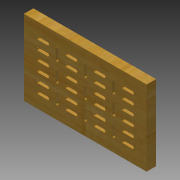
# Autodesk Inventor part: suporte
Saved by Autodesk Inventor 2014 (Build 180170000, 170)
## iProperties
Created: 2015-05-28
Part Number: suporte
Material: Generic
Document SubType Name: Modeling
Designer: Gabriel
Density: 1 g/cm^3
Appearance: Default
Author: Gabriel
Autodesk Inventor part; units mm, degrees
ref_plane "YZ Plane" through (0, 0, 0) normal (1, 0, 0) x (0, 1, 0)
ref_plane "XZ Plane" through (0, 0, 0) normal (0, 1, 0) x (-1, 0, 0)
ref_plane "XY Plane" through (0, 0, 0) normal (0, 0, 1) x (1, 0, 0)
sketch "Sketch1" plane through (0, 0, 0) normal (0, 1, 0) x (-1, 0, 0)
  line L0 (0, 0) -> (130, 0)
  line L1 (130, 0) -> (130, 80)
  line L2 (130, 80) -> (0, 80)
  line L3 (0, 80) -> (0, 0)
  line L4 (0, 0) -> (0, 20)
  line L5 (130, 0) -> (110, 0)
  line L6 (130, 80) -> (110, 80)
  line L7 (0, 80) -> (0, 55)
  line L8 (23.5, 55) -> (25, 55)
  line L9 (25, 55) -> (23.5, 55) construction
  line L10 (25, 56.5) -> (15, 56.5)
  line L11 (15, 53.5) -> (25, 53.5)
  arc A0 (25, 53.5) -> (25, 56.5) centre (25, 55) ccw
  arc A1 (15, 56.5) -> (15, 53.5) centre (15, 55) ccw
  line L12 (20, 25) -> (15, 25)
  line L13 (15, 25) -> (25, 25) construction
  line L14 (15, 23.5) -> (25, 23.5)
  line L15 (25, 26.5) -> (15, 26.5)
  arc A2 (15, 26.5) -> (15, 23.5) centre (15, 25) ccw
  arc A3 (25, 23.5) -> (25, 26.5) centre (25, 25) ccw
  line L16 (20, 55) -> (20, 45)
  line L17 (25, 45) -> (15, 45) construction
  line L18 (25, 46.5) -> (15, 46.5)
  line L19 (15, 43.5) -> (25, 43.5)
  arc A4 (25, 43.5) -> (25, 46.5) centre (25, 45) ccw
  arc A5 (15, 46.5) -> (15, 43.5) centre (15, 45) ccw
  line L20 (25, 35) -> (15, 35) construction
  line L21 (25, 36.5) -> (15, 36.5)
  line L22 (15, 33.5) -> (25, 33.5)
  arc A6 (25, 33.5) -> (25, 36.5) centre (25, 35) ccw
  arc A7 (15, 36.5) -> (15, 33.5) centre (15, 35) ccw
  line L23 (20, 55) -> (20, 65)
  line L24 (20, 65) -> (20, 66.5)
  line L25 (25, 65) -> (15, 65) construction
  line L26 (25, 66.5) -> (15, 66.5)
  line L27 (15, 63.5) -> (25, 63.5)
  arc A8 (25, 63.5) -> (25, 66.5) centre (25, 65) ccw
  arc A9 (15, 66.5) -> (15, 63.5) centre (15, 65) ccw
  line L28 (25, 15) -> (15, 15) construction
  line L29 (25, 16.5) -> (15, 16.5)
  line L30 (15, 13.5) -> (25, 13.5)
  arc A10 (25, 13.5) -> (25, 16.5) centre (25, 15) ccw
  arc A11 (15, 16.5) -> (15, 13.5) centre (15, 15) ccw
  line L31 (20, 80) -> (35, 80)
  line L32 (35, 80) -> (50, 80)
  line L33 (50, 80) -> (70, 80)
  line L34 (70, 80) -> (90, 80)
  line L35 (46.5, 55) -> (45, 55)
  line L36 (45, 55) -> (46.5, 55) construction
  line L37 (45, 56.5) -> (55, 56.5)
  line L38 (55, 53.5) -> (45, 53.5)
  arc A12 (45, 56.5) -> (45, 53.5) centre (45, 55) ccw
  arc A13 (55, 53.5) -> (55, 56.5) centre (55, 55) ccw
  line L39 (50, 25) -> (55, 25)
  line L40 (55, 25) -> (45, 25) construction
  line L41 (55, 23.5) -> (45, 23.5)
  line L42 (45, 26.5) -> (55, 26.5)
  arc A14 (55, 23.5) -> (55, 26.5) centre (55, 25) ccw
  arc A15 (45, 26.5) -> (45, 23.5) centre (45, 25) ccw
  line L43 (45, 45) -> (55, 45) construction
  line L44 (45, 46.5) -> (55, 46.5)
  line L45 (55, 43.5) -> (45, 43.5)
  arc A16 (45, 46.5) -> (45, 43.5) centre (45, 45) ccw
  arc A17 (55, 43.5) -> (55, 46.5) centre (55, 45) ccw
  line L46 (45, 35) -> (55, 35) construction
  line L47 (45, 36.5) -> (55, 36.5)
  line L48 (55, 33.5) -> (45, 33.5)
  arc A18 (45, 36.5) -> (45, 33.5) centre (45, 35) ccw
  arc A19 (55, 33.5) -> (55, 36.5) centre (55, 35) ccw
  line L49 (45, 65) -> (55, 65) construction
  line L50 (45, 66.5) -> (55, 66.5)
  line L51 (55, 63.5) -> (45, 63.5)
  arc A20 (45, 66.5) -> (45, 63.5) centre (45, 65) ccw
  arc A21 (55, 63.5) -> (55, 66.5) centre (55, 65) ccw
  line L52 (45, 15) -> (55, 15) construction
  line L53 (45, 16.5) -> (55, 16.5)
  line L54 (55, 13.5) -> (45, 13.5)
  arc A22 (45, 16.5) -> (45, 13.5) centre (45, 15) ccw
  arc A23 (55, 13.5) -> (55, 16.5) centre (55, 15) ccw
  line L55 (50, 80) -> (65, 80)
  line L56 (65, 80) -> (80, 80)
  arc A24 (75, 56.5) -> (75, 53.5) centre (75, 55) ccw
  line L57 (83.5, 55) -> (85, 55)
  line L58 (85, 55) -> (83.5, 55) construction
  line L59 (75, 53.5) -> (85, 53.5)
  arc A25 (85, 53.5) -> (85, 56.5) centre (85, 55) ccw
  arc A26 (85, 23.5) -> (85, 26.5) centre (85, 25) ccw
  arc A27 (75, 26.5) -> (75, 23.5) centre (75, 25) ccw
  line L60 (75, 23.5) -> (85, 23.5)
  line L61 (75, 43.5) -> (85, 43.5)
  line L62 (85, 45) -> (75, 45) construction
  arc A28 (75, 46.5) -> (75, 43.5) centre (75, 45) ccw
  line L63 (85, 46.5) -> (75, 46.5)
  arc A29 (85, 43.5) -> (85, 46.5) centre (85, 45) ccw
  line L64 (80, 25) -> (75, 25)
  line L65 (85, 36.5) -> (75, 36.5)
  arc A30 (85, 33.5) -> (85, 36.5) centre (85, 35) ccw
  line L66 (85, 35) -> (75, 35) construction
  line L67 (75, 33.5) -> (85, 33.5)
  arc A31 (75, 36.5) -> (75, 33.5) centre (75, 35) ccw
  line L68 (85, 26.5) -> (75, 26.5)
  line L69 (75, 25) -> (85, 25) construction
  line L70 (85, 56.5) -> (75, 56.5)
  line L71 (75, 63.5) -> (85, 63.5)
  line L72 (85, 65) -> (75, 65) construction
  line L73 (85, 66.5) -> (75, 66.5)
  arc A32 (75, 66.5) -> (75, 63.5) centre (75, 65) ccw
  arc A33 (85, 63.5) -> (85, 66.5) centre (85, 65) ccw
  line L74 (85, 16.5) -> (75, 16.5)
  line L75 (85, 15) -> (75, 15) construction
  arc A34 (75, 16.5) -> (75, 13.5) centre (75, 15) ccw
  arc A35 (85, 13.5) -> (85, 16.5) centre (85, 15) ccw
  line L76 (75, 13.5) -> (85, 13.5)
  line L77 (80, 80) -> (95, 80)
  line L78 (95, 0) -> (110, 0)
  arc A36 (105, 56.5) -> (105, 53.5) centre (105, 55) ccw
  arc A37 (105, 66.5) -> (105, 63.5) centre (105, 65) ccw
  arc A38 (115, 63.5) -> (115, 66.5) centre (115, 65) ccw
  line L79 (106.5, 55) -> (105, 55)
  line L80 (105, 55) -> (106.5, 55) construction
  line L81 (115, 63.5) -> (105, 63.5)
  line L82 (105, 66.5) -> (115, 66.5)
  line L83 (105, 65) -> (115, 65) construction
  line L84 (105, 56.5) -> (115, 56.5)
  arc A39 (115, 53.5) -> (115, 56.5) centre (115, 55) ccw
  line L85 (115, 23.5) -> (105, 23.5)
  arc A40 (105, 16.5) -> (105, 13.5) centre (105, 15) ccw
  line L86 (105, 16.5) -> (115, 16.5)
  line L87 (105, 15) -> (115, 15) construction
  line L88 (115, 13.5) -> (105, 13.5)
  arc A41 (115, 13.5) -> (115, 16.5) centre (115, 15) ccw
  line L89 (115, 53.5) -> (105, 53.5)
  line L90 (105, 46.5) -> (115, 46.5)
  line L91 (105, 45) -> (115, 45) construction
  arc A42 (105, 46.5) -> (105, 43.5) centre (105, 45) ccw
  line L92 (115, 43.5) -> (105, 43.5)
  arc A43 (115, 43.5) -> (115, 46.5) centre (115, 45) ccw
  arc A44 (105, 26.5) -> (105, 23.5) centre (105, 25) ccw
  arc A45 (115, 23.5) -> (115, 26.5) centre (115, 25) ccw
  line L93 (110, 25) -> (115, 25)
  line L94 (115, 25) -> (105, 25) construction
  line L95 (105, 26.5) -> (115, 26.5)
  line L96 (115, 33.5) -> (105, 33.5)
  line L97 (105, 35) -> (115, 35) construction
  arc A46 (115, 33.5) -> (115, 36.5) centre (115, 35) ccw
  line L98 (105, 36.5) -> (115, 36.5)
  arc A47 (105, 36.5) -> (105, 33.5) centre (105, 35) ccw
  line L99 (33.5, 65) -> (33.5, 55)
  line L100 (36.5, 55) -> (36.5, 65)
  arc A48 (36.5, 65) -> (33.5, 65) centre (35, 65) ccw
  arc A49 (33.5, 55) -> (36.5, 55) centre (35, 55) ccw
  line L101 (65, 65) -> (65, 55) construction
  line L102 (63.5, 65) -> (63.5, 55)
  line L103 (66.5, 55) -> (66.5, 65)
  arc A50 (66.5, 65) -> (63.5, 65) centre (65, 65) ccw
  arc A51 (63.5, 55) -> (66.5, 55) centre (65, 55) ccw
  line L104 (65, 45) -> (65, 35) construction
  line L105 (63.5, 45) -> (63.5, 35)
  line L106 (66.5, 35) -> (66.5, 45)
  arc A52 (66.5, 45) -> (63.5, 45) centre (65, 45) ccw
  arc A53 (63.5, 35) -> (66.5, 35) centre (65, 35) ccw
  line L107 (65, 25) -> (65, 15) construction
  line L108 (63.5, 25) -> (63.5, 15)
  line L109 (66.5, 15) -> (66.5, 25)
  arc A54 (66.5, 25) -> (63.5, 25) centre (65, 25) ccw
  arc A55 (63.5, 15) -> (66.5, 15) centre (65, 15) ccw
  line L110 (95, 65) -> (95, 55) construction
  line L111 (93.5, 65) -> (93.5, 55)
  line L112 (96.5, 55) -> (96.5, 65)
  arc A56 (96.5, 65) -> (93.5, 65) centre (95, 65) ccw
  arc A57 (93.5, 55) -> (96.5, 55) centre (95, 55) ccw
  line L113 (95, 45) -> (95, 35) construction
  line L114 (93.5, 45) -> (93.5, 35)
  line L115 (96.5, 35) -> (96.5, 45)
  arc A58 (96.5, 45) -> (93.5, 45) centre (95, 45) ccw
  arc A59 (93.5, 35) -> (96.5, 35) centre (95, 35) ccw
  line L116 (95, 25) -> (95, 15) construction
  line L117 (93.5, 25) -> (93.5, 15)
  line L118 (96.5, 15) -> (96.5, 25)
  arc A60 (96.5, 25) -> (93.5, 25) centre (95, 25) ccw
  arc A61 (93.5, 15) -> (96.5, 15) centre (95, 15) ccw
  line L119 (20, 55) -> (20, 66.5)
  line L120 (20, 75) -> (20, 80)
  line L121 (33.5, 45) -> (33.5, 35)
  line L122 (36.5, 35) -> (36.5, 45)
  arc A62 (36.5, 45) -> (33.5, 45) centre (35, 45) ccw
  arc A63 (33.5, 35) -> (36.5, 35) centre (35, 35) ccw
  line L123 (35, 25) -> (35, 15) construction
  line L124 (33.5, 25) -> (33.5, 15)
  line L125 (36.5, 15) -> (36.5, 25)
  arc A64 (36.5, 25) -> (33.5, 25) centre (35, 25) ccw
  arc A65 (33.5, 15) -> (36.5, 15) centre (35, 15) ccw
  line L126 (35, 45) -> (35, 43.5) construction
  line L127 (35, 36.5) -> (35, 35) construction
  line L128 (35, 56.5) -> (35, 55) construction
  point P0 (20, 0)
  point P1 (130, 20)
  point P2 (130, 60)
  point P3 (13.5, 55)
  point P4 (20, 45)
  point P5 (20, 35)
  point P6 (20, 65)
  point P7 (20, 15)
  point P8 (56.5, 55)
  point P9 (73.5, 55)
  point P10 (80, 65)
  point P11 (110, 15)
  point P12 (110, 65)
  point P13 (116.5, 55)
  point P14 (35, 60)
  point P15 (65, 60)
  point P16 (65, 40)
  point P17 (65, 20)
  point P18 (95, 60)
  point P19 (95, 40)
  point P20 (95, 20)
  point P21 (35, 40)
  point P22 (35, 20)
  dimension "d0" = 130
  dimension "d1" = 80
  dimension "d5" = 20
  dimension "d7" = 20
  dimension "d10" = 20
  dimension "d14" = 5
  dimension "d17" = 10
  dimension "d18" = 3
  dimension "d28" = 25
  dimension "d29" = 5
  dimension "d30" = 10
  dimension "d32" = 25
  dimension "d37" = 10
  dimension "d38" = 3
  dimension "d40" = 3
  dimension "d41" = 10
  dimension "d42" = 10
  dimension "d44" = 10
  dimension "d45" = 3
  dimension "d51" = 15
  dimension "d52" = 15
  dimension "d53" = 15
  dimension "d54" = 15
  dimension "d55" = 3
  dimension "d63" = 3
  dimension "d64" = 3
  dimension "d65" = 3
  dimension "d66" = 3
  dimension "d67" = 3
  dimension "d68" = 3
  dimension "d69" = 3
  dimension "d70" = 3
  constraints: 314 end point, 140 point on circle, 66 centre point, 60 tangent, 23 point on line, 19 parallel, 13 midpoint, 2 horizontal, 2 vertical, 1 perpendicular, 10 other
  measures "d0" distance of L3.start L1.end
  measures "d1" distance of L3.start L0.start
  measures "d5" distance of L0.end L5.end
  measures "d7" distance of L1.end L6.end
  measures "d10" distance of L16.start L7.end
  measures "d14" distance of L16.start L8.end
  measures "d17" distance of L8.end A1.centre
  measures "d18" diameter of A1
  measures "d28" distance of L12.start point (20, 0)
  measures "d29" distance of L12.start L12.end
  measures "d30" distance of L12.end L13.end
  measures "d32" distance of L16.start L31.start
  measures "d37" distance of L16.start L16.end
  measures "d38" diameter of A5
  measures "d40" diameter of A7
  measures "d41" distance of L16.start L23.end
  measures "d42" distance of L120.start L23.end
  measures "d44" distance of L25.start L25.end
  measures "d45" diameter of A9
  measures "d51" distance of L32.end L55.end
  measures "d52" distance of L55.end L56.end
  measures "d53" distance of L56.end L77.end
  measures "d54" distance of L78.start L78.end
  measures "d55" diameter of A49
  measures "d63" diameter of A51
  measures "d64" diameter of A53
  measures "d65" diameter of A55
  measures "d66" diameter of A57
  measures "d67" diameter of A59
  measures "d68" diameter of A61
  measures "d69" diameter of A63
  measures "d70" diameter of A65
extrude "Extrusion3" add sketch "Sketch1" along normal blind 10
body "Solid3"
